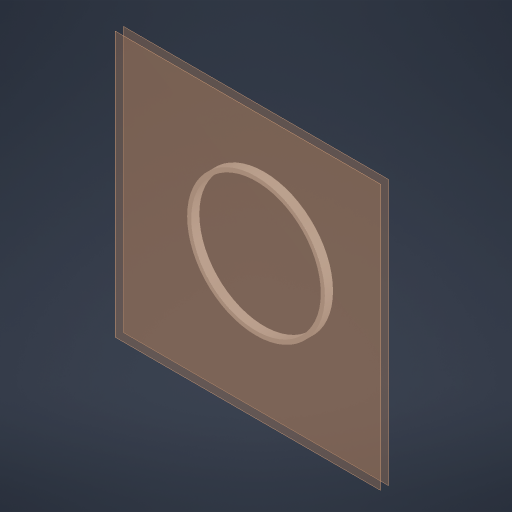
# Autodesk Inventor part: LedStrip
Saved by Autodesk Inventor 2023.1 (Build 271208000, 208)
## iProperties
Created: 2023-08-24
Part Number: LedStrip
Material: Generic
Document SubType Name: Modeling
Designer: washichi
Density: 1 g/cm^3
Appearance: Default
Author: washichi
Autodesk Inventor part; units mm, degrees
ref_plane "YZ Plane" through (0, 0, 0) normal (1, 0, 0) x (0, 1, 0)
ref_plane "XZ Plane" through (0, 0, 0) normal (0, 1, 0) x (-1, 0, 0)
ref_plane "XY Plane" through (0, 0, 0) normal (0, 0, 1) x (1, 0, 0)
ref_plane "Work Plane1" through (-9.4462, 53.9314, -71.7677) normal (0, 0, 1) x (1, 0, 0)
ref_plane "Work Plane2" through (-9.4462, 53.9314, -81.7677) normal (0, 0, 1) x (1, 0, 0)
sketch "Sketch1" plane through (-9.4462, 53.9314, -81.7677) normal (0, 0, 1) x (1, 0, 0)
  circle A0 centre (0, 0) radius 79.5775
  circle A1 centre (0, 0) radius 84.5775
  point P0 (9.4462, -53.9314)
  dimension "d0" = 159.155
  dimension "d1" = 5
  constraints: 2 centre point
  measures "d0" diameter of A0
  measures "d1" radial gap between concentric circles of A0 A1
extrude "Extrusion1" add sketch "Sketch1" against normal blind 10
body "Solid1"
